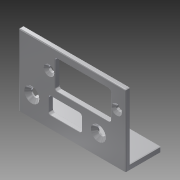
# Autodesk Inventor part: Držák
Saved by Autodesk Inventor 2013 (Build 170138000, 138)
## iProperties
Created: 2013-02-15
Part Number: Držák
Material: Hliník 6061-AHC
Document SubType Name: Modeling
Designer: jirka1
Density: 0.9983 g/cm^3
Author: jirka1
Autodesk Inventor part; units mm, degrees
ref_plane "YZ Plane" through (0, 0, 0) normal (1, 0, 0) x (0, 1, 0)
ref_plane "XZ Plane" through (0, 0, 0) normal (0, 1, 0) x (-1, 0, 0)
ref_plane "XY Plane" through (0, 0, 0) normal (0, 0, 1) x (1, 0, 0)
sketch "Náčrt1" plane through (0, 0, 0) normal (1, 0, 0) x (0, 1, 0)
  line L0 (0, 0) -> (0, 30)
  line L1 (0, 0) -> (30, 0) construction
  line L2 (0, 30) -> (2, 30)
  line L3 (2, 30) -> (2, 2)
  line L4 (2, 2) -> (15, 2)
  line L5 (15, 2) -> (15, 0)
  line L6 (15, 0) -> (0, 0)
  dimension "d0" = 30
  dimension "d1" = 90
  dimension "d2" = 2
  dimension "d3" = 28
  dimension "d4" = 13
  constraints: 14 end point, 4 parallel, 2 perpendicular, 1 horizontal, 1 vertical
  measures "d0" distance of L0.start L0.end
  measures "d1" angle of L1 L0
  measures "d2" distance of L0.end L2.end
  measures "d3" distance of L2.end L3.end
  measures "d4" distance of L3.end L4.end
extrude "Vysunutí1" add sketch "Náčrt1" along normal blind 45
hole "Díra1" at (5.5, 0, 8.5) direction (0, 1, 0) diameter 3.4 end through all countersink diameter 6.3 countersink angle 90 clearance for "Strojní šroub se zápustnou hlavou" size "M3" standard "Ansi M metrický profil"
hole "Díra2" at (33.5, 0, 8.5) direction (0, 1, 0) diameter 3.4 end through all countersink diameter 6.3 countersink angle 90 clearance for "Strojní šroub se zápustnou hlavou" size "M3" standard "Ansi M metrický profil"
sketch "Náčrt3" plane through (0, 0, 0) normal (0, -1, 0) x (1, 0, 0)
  line L0 (13.5, 5) -> (25.5, 5)
  line L1 (26.5, 6) -> (26.5, 11)
  line L2 (25.5, 12) -> (13.5, 12)
  line L3 (12.5, 11) -> (12.5, 6)
  line L4 (12.5, 5) -> (26.5, 12) construction
  line L5 (26.5, 5) -> (12.5, 12) construction
  arc A0 (13.5, 12) -> (12.5, 11) centre (13.5, 11) ccw
  arc A1 (26.5, 11) -> (25.5, 12) centre (25.5, 11) ccw
  arc A2 (25.5, 5) -> (26.5, 6) centre (25.5, 6) ccw
  arc A3 (12.5, 6) -> (13.5, 5) centre (13.5, 6) ccw
  point P0 (19.5, 8.5)
  dimension "d29" = 14
  dimension "d30" = 7
  dimension "d31" = 1
  constraints: 12 end point, 8 point on circle, 8 point on line, 8 tangent, 4 centre point, 3 equal radius, 2 midpoint, 2 parallel, 1 horizontal, 1 perpendicular
  measures "d29" distance of L5.end L4.end
  measures "d30" distance of L4.end L5.start
  measures "d31" radius of A0
extrude "Vysunutí2" cut sketch "Náčrt3" against normal blind 2
hole "Díra3" at (12.75, 0, 21) direction (0, 1, 0) diameter 2.4 end through all countersink diameter 4.4 countersink angle 90 clearance for "Strojní šroub se zápustnou hlavou" size "M2" standard "Ansi M metrický profil"
hole "Díra4" at (41.25, 0, 21) direction (0, 1, 0) diameter 2.4 end through all countersink diameter 4.4 countersink angle 90 clearance for "Strojní šroub se zápustnou hlavou" size "M2" standard "Ansi M metrický profil"
sketch "Náčrt2" plane through (0, 0, 0) normal (0, -1, 0) x (1, 0, 0)
  line L0 (45, 30) -> (45, 0) projected
  line L1 (-5, 2) -> (45, 2)
  line L2 (16.25, 15) -> (37.75, 15)
  line L3 (38.75, 16) -> (38.75, 26)
  line L4 (37.75, 27) -> (16.25, 27)
  line L5 (15.25, 26) -> (15.25, 16)
  line L6 (15.25, 15) -> (38.75, 27) construction
  line L7 (38.75, 15) -> (15.25, 27) construction
  arc A0 (16.25, 27) -> (15.25, 26) centre (16.25, 26) ccw
  arc A1 (38.75, 26) -> (37.75, 27) centre (37.75, 26) ccw
  arc A2 (37.75, 15) -> (38.75, 16) centre (37.75, 16) ccw
  arc A3 (15.25, 16) -> (16.25, 15) centre (16.25, 16) ccw
  point P0 (27, 21)
  dimension "d54" = 23.5
  dimension "d55" = 12
  dimension "d58" = 1
  constraints: 14 end point, 9 point on line, 8 point on circle, 8 tangent, 4 centre point, 3 equal radius, 2 midpoint, 2 parallel, 2 perpendicular, 1 horizontal
  measures "d54" distance of L7.end L6.end
  measures "d55" distance of L6.end L7.start
  measures "d58" radius of A0
extrude "Vysunutí3" cut sketch "Náčrt2" against normal blind 2
fillet "Zaoblení1" radius 0.4 13 edges at (22.5, 0, 30) (22.5, 2, 30) (45, 0, 15) (45, 2, 16) (45, 1, 30) (45, 8.5, 2) (22.5, 15, 2) (45, 15, 1) (0, 0, 15) (0, 1, 30) (0, 2, 16) (0, 8.5, 2) (0, 15, 1)
fillet "Zaoblení2" radius 0.2 32 edges at (38.4571, 0, 26.7071) (38.75, 0, 21) (38.4571, 0, 15.2929) (27, 0, 15) (15.5429, 0, 15.2929) (15.25, 0, 21) (15.5429, 0, 26.7071) (27, 0, 27) (26.2071, 0, 11.7071) (26.5, 0, 8.5) (26.2071, 0, 5.2929) (19.5, 0, 5) (12.7929, 0, 5.2929) (12.5, 0, 8.5) (12.7929, 0, 11.7071) (19.5, 0, 12) (15.5429, 2, 26.7071) (15.25, 2, 21) (15.5429, 2, 15.2929) (27, 2, 15) (38.4571, 2, 15.2929) (38.75, 2, 21) (38.4571, 2, 26.7071) (27, 2, 27) (12.7929, 2, 11.7071) (12.5, 2, 8.5) (12.7929, 2, 5.2929) (19.5, 2, 5) (26.2071, 2, 5.2929) (26.5, 2, 8.5) (26.2071, 2, 11.7071) (19.5, 2, 12)
